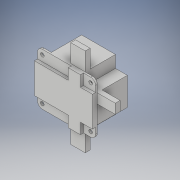
# Autodesk Inventor part: h bridge
Saved by Autodesk Inventor 2019.3 (Build 233278000, 278)
## iProperties
Created: 2019-06-10
Part Number: h bridge
Material: Generic
Document SubType Name: Modeling
Designer: Frienddo
Density: 1 g/cm^3
Appearance: Default
Author: Frienddo
Autodesk Inventor part; units mm, degrees
ref_plane "YZ Plane" through (0, 0, 0) normal (1, 0, 0) x (0, 1, 0)
ref_plane "XZ Plane" through (0, 0, 0) normal (0, 1, 0) x (-1, 0, 0)
ref_plane "XY Plane" through (0, 0, 0) normal (0, 0, 1) x (1, 0, 0)
sketch "Sketch1" plane through (0, 0, 0) normal (0, 0, 1) x (1, 0, 0)
  line L0 (20, -21.5) -> (-20, -21.5)
  line L1 (-24, -17.5) -> (-24, 17.5)
  line L2 (-20, 21.5) -> (20, 21.5)
  line L3 (24, 17.5) -> (24, -17.5)
  line L4 (24, -21.5) -> (-24, 21.5) construction
  line L5 (-24, -21.5) -> (24, 21.5) construction
  arc A0 (24, 17.5) -> (20, 21.5) centre (20, 17.5) ccw
  arc A1 (-20, 21.5) -> (-24, 17.5) centre (-20, 17.5) ccw
  arc A2 (-24, -17.5) -> (-20, -21.5) centre (-20, -17.5) ccw
  arc A3 (20, -21.5) -> (24, -17.5) centre (20, -17.5) ccw
  circle A4 centre (-20, 17.5) radius 1.5
  circle A5 centre (20, 17.5) radius 1.5
  circle A6 centre (20, -17.5) radius 1.5
  circle A7 centre (-20, -17.5) radius 1.5
  point P0 (0, 0)
  dimension "d0" = 48
  dimension "d1" = 43
  dimension "d2" = 4
  dimension "d3" = 3
  dimension "d4" = 3
  dimension "d5" = 3
  dimension "d6" = 3
  constraints: 12 end point, 8 centre point, 8 point on circle, 8 point on line, 8 tangent, 4 coincident, 3 equal radius, 2 midpoint, 2 parallel, 1 horizontal, 1 perpendicular
  measures "d0" distance of L4.end L5.end
  measures "d1" distance of L5.start L4.end
  measures "d2" radius of A0
  measures "d3" diameter of A4
  measures "d4" diameter of A5
  measures "d5" diameter of A6
  measures "d6" diameter of A7
extrude "Extrusion1" add sketch "Sketch1" along normal blind 1.5
sketch "Sketch2" plane through (0, 0, 1.5) normal (0, 0, 1) x (1, 0, 0)
  line L0 (-24, 17.5) -> (-24, -17.5) projected
  line L1 (24, -12.5) -> (-24, -12.5)
  line L2 (-24, -12.5) -> (-24, 12.5)
  line L3 (-24, 12.5) -> (24, 12.5)
  line L4 (24, 12.5) -> (24, -12.5)
  line L5 (24, -12.5) -> (-24, 12.5) construction
  line L6 (-24, -12.5) -> (24, 12.5) construction
  line L7 (20, 21.5) -> (-20, 21.5) projected
  line L8 (-20, -21.5) -> (20, -21.5) projected
  line L9 (14, 21.5) -> (4, 21.5)
  line L10 (4, 21.5) -> (4, -21.5)
  line L11 (4, -21.5) -> (14, -21.5)
  line L12 (14, -21.5) -> (14, 21.5)
  point P0 (0, 0)
  dimension "d9" = 25
  dimension "d10" = 10
  dimension "d11" = 10
  constraints: 20 end point, 4 parallel, 3 point on line, 2 horizontal, 2 midpoint, 2 perpendicular
  measures "d9" distance between parallel lines of L1 L3
  measures "d10" distance between parallel lines of L4 L12
  measures "d11" distance between parallel lines of L12 L10
extrude "Extrusion2" add sketch "Sketch2" along normal blind 2.5
sketch "Sketch3" plane through (0, 0, 0) normal (0, 0, -1) x (-1, 0, 0)
  line L0 (23.8696, 11.5) -> (-23.8696, 11.5)
  line L1 (-23.8696, 11.5) -> (-23.8696, -11.5)
  line L2 (-23.8696, -11.5) -> (23.8696, -11.5)
  line L3 (23.8696, -11.5) -> (23.8696, 11.5)
  line L4 (23.8696, 11.5) -> (-23.8696, -11.5) construction
  line L5 (-23.8696, 11.5) -> (23.8696, -11.5) construction
  line L6 (20, -21.5) -> (-20, -21.5) projected
  line L7 (14, 21.5) -> (-14, 21.5)
  line L8 (-14, 21.5) -> (-14, -21.5)
  line L9 (-14, -21.5) -> (14, -21.5)
  line L10 (14, -21.5) -> (14, 21.5)
  line L11 (14, 21.5) -> (-14, -21.5) construction
  line L12 (-14, 21.5) -> (14, -21.5) construction
  line L13 (-24, -17.5) -> (-24, 17.5) projected
  point P0 (0, 0)
  dimension "d14" = 10
  dimension "d15" = 10
  constraints: 24 end point, 4 midpoint, 4 parallel, 2 horizontal, 2 perpendicular, 1 point on line
  measures "d14" distance between parallel lines of L13 L8
  measures "d15" distance between parallel lines of L6 L2
extrude "Extrusion3" add sketch "Sketch3" along normal blind 25
sketch "Sketch4" plane through (20, -21.5, 0) normal (0, -1, 0) x (1, 0, 0)
  line L0 (-6, 0) -> (0, 0) projected
  line L1 (-6, 0) -> (-18, 0)
  line L2 (-18, 0) -> (-18, -4)
  line L3 (-18, -4) -> (-6, -4)
  line L4 (-6, -4) -> (-6, 0)
  point P0 (-20, 0)
  dimension "d18" = 12
  dimension "d19" = 4
  constraints: 8 end point, 2 parallel, 1 horizontal, 1 perpendicular
  measures "d18" distance of L3.end L2.end
  measures "d19" distance between parallel lines of L1 L3
extrude "Extrusion4" add sketch "Sketch4" along normal blind 15
mirror "Mirror1" about plane through (0, 0, 0) normal (0, 1, 0) of "Extrusion4"
sketch "Sketch5" plane through (23.8696, -11.5, 0) normal (1, 0, 0) x (0, 0, -1)
  line L0 (0, 23) -> (25, 23) projected
  line L1 (0, 23) -> (4, 23)
  line L2 (4, 23) -> (4, 15)
  line L3 (4, 15) -> (0, 15)
  line L4 (0, 15) -> (0, 23)
  point P0 (0, 11.5)
  dimension "d22" = 4
  dimension "d23" = 8
  constraints: 8 end point, 2 parallel, 1 horizontal, 1 perpendicular
  measures "d22" distance of L2.end L3.end
  measures "d23" distance of L1.end L2.end
extrude "Extrusion5" add sketch "Sketch5" along normal blind 15
body "Solid1"
